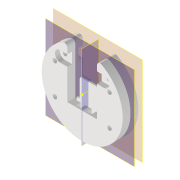
# Autodesk Inventor part: Matchboxscope_layer_ikealamp
Saved by Autodesk Inventor 2022 (Build 260153000, 153)
## iProperties
Created: 2022-04-02
Part Number: Matchboxscope_layer_ikealamp
Material: Generic
Document SubType Name: Modeling
Designer: Prakash Lab
Density: 1 g/cm^3
Appearance: Default
Author: Prakash Lab
Autodesk Inventor part; units mm, degrees
ref_plane "YZ Plane" through (0, 0, 0) normal (1, 0, 0) x (0, 1, 0)
ref_plane "XZ Plane" through (0, 0, 0) normal (0, 1, 0) x (-1, 0, 0)
ref_plane "XY Plane" through (0, 0, 0) normal (0, 0, 1) x (1, 0, 0)
ref_plane "Work Plane1" through (0, 0, 0) normal (0, 0, 1) x (1, 0, 0)
sketch "Sketch1" plane through (0, 0, 0) normal (0, 0, 1) x (1, 0, 0)
  circle A0 centre (0, 0) radius 25.9979 projected
  circle A1 centre (-9.4998, -11.0022) radius 2.6601 projected
  circle A2 centre (0.0001, -0.0022) radius 3.8801 projected
  circle A3 centre (0.0001, -0.0022) radius 6.7754 projected
  circle A4 centre (0.0001, -0.0022) radius 10
  point P0 (0, 0)
  dimension "d17" = 20
  constraints: 1 centre point, 1 coincident
  measures "d17" diameter of A4
extrude "Extrusion1" add sketch "Sketch1" along normal blind 10 contours A0 | A1 | A2 | A3 | A4
ref_plane "Arbeitsebene4" through (0, 0, 5) normal (0, 0, -1) x (-1, 0, 0)
sketch "Skizze22" plane through (0, 0, 10) normal (0, 0, 1) x (1, 0, 0)
  circle A0 centre (0, 0) radius 25.9979 projected
  line L0 (-9.5, 60.9958) -> (9.5, 60.9958)
  line L1 (9.5, 60.9958) -> (9.5, -9)
  line L2 (9.5, -9) -> (-9.5, -9)
  line L3 (-9.5, -9) -> (-9.5, 60.9958)
  line L4 (-9.5, 60.9958) -> (9.5, -9) construction
  line L5 (9.5, 60.9958) -> (-9.5, -9) construction
  point P0 (0, 0)
  point P1 (0, 25.9979)
  point P2 (2.05, -9)
  dimension "d82" = 19
  constraints: 12 end point, 2 midpoint, 2 parallel, 1 horizontal, 1 perpendicular, 1 point on line, 1 vertical alignment, 2 other
  measures "d82" distance of L1.end L2.end
extrude "Extrusion16" cut sketch "Skizze22" against normal blind 10 contours L1 L2 L3 A0 | A0 L3 L0 L1 picked at (-1.0778, 2.5987)
sketch "Skizze23" plane through (0, 0, 5) normal (0, 0, -1) x (-1, 0, 0)
  line L0 (-5.5222, 4.15) -> (-5.3125, 4.7) projected
  line L1 (-5.3125, 4.7) -> (5.3352, 4.7) projected
  line L2 (5.3352, 4.7) -> (5.5222, 4.15) projected
  line L3 (5.5222, 4.15) -> (5.7, 3.9722) projected
  line L4 (5.7, 3.9722) -> (5.7, -4) projected
  line L5 (4.85, -4) -> (5.7, -4) projected
  arc A0 (4.05, -3.2) -> (4.85, -4) centre (4.85, -3.2) ccw projected
  line L6 (4.05, -3.2) -> (4.05, 1.7) projected
  line L7 (4.05, 1.7) -> (2.85, 1.7) projected
  line L8 (2.85, -3.2) -> (2.85, 1.7) projected
  arc A1 (2.05, -4) -> (2.85, -3.2) centre (2.05, -3.2) ccw projected
  line L9 (-2.05, -4) -> (2.05, -4) projected
  arc A2 (-2.85, -3.2) -> (-2.05, -4) centre (-2.05, -3.2) ccw projected
  line L10 (-2.85, -3.2) -> (-2.85, 1.7) projected
  line L11 (-2.85, 1.7) -> (-4.05, 1.7) projected
  line L12 (-4.05, -3.2) -> (-4.05, 1.7) projected
  arc A3 (-4.85, -4) -> (-4.05, -3.2) centre (-4.85, -3.2) ccw projected
  line L13 (-5.7, -4) -> (-4.85, -4) projected
  line L14 (-5.7, -4) -> (-5.7, 3.9722) projected
  line L15 (-5.7, 3.9722) -> (-5.5222, 4.15) projected
  line L16 (5.7, -4) -> (5.7, -7) projected
  line L17 (5.7, -7) -> (7.5, -7) projected
  line L18 (7.5, -7) -> (7.5, -9) projected
  line L19 (7.5, -9) -> (4.85, -9) projected
  line L20 (4.85, -6) -> (4.85, -9) projected
  line L21 (4.85, -4) -> (4.85, -6) projected
  line L22 (4.85, -4) -> (5.7, -4) projected
  line L23 (-5.7, -7) -> (-5.7, -4) projected
  line L24 (-5.7, -4) -> (-4.85, -4) projected
  line L25 (-4.85, -4) -> (-4.85, -6) projected
  line L26 (-4.85, -6) -> (-4.85, -9) projected
  line L27 (-4.85, -9) -> (-7.5, -9) projected
  line L28 (-7.5, -9) -> (-7.5, -7) projected
  line L29 (-7.5, -7) -> (-5.7, -7) projected
  line L30 (-4.85, -9) -> (4.85, -9)
  constraints: 2 end point, 1 horizontal
extrude "Extrusion17" add sketch "Skizze23" along normal mid plane 1.9
sketch "Skizze24" plane through (0, 0, 5.95) normal (0, 0, -1) x (1, 0, 0)
  line L0 (2.85, 3.2) -> (2.85, -1.7) projected
  line L1 (2.85, -1.7) -> (4.05, -1.7) projected
  line L2 (4.05, 3.2) -> (4.05, -1.7) projected
  arc A0 (4.85, 4) -> (4.05, 3.2) centre (4.85, 3.2) ccw projected
  line L3 (4.85, 4) -> (4.85, 6) projected
  arc A1 (2.85, 3.2) -> (2.05, 4) centre (2.05, 3.2) ccw projected
  line L4 (2.05, 4) -> (2.05, 6) projected
  line L5 (4.85, 6) -> (4.85, 9) projected
  line L6 (2.05, 6) -> (2.05, 9) projected
  line L7 (9.5, 9) -> (-9.5, 9) projected
  line L8 (-2.05, 6) -> (-2.05, 9) projected
  line L9 (-4.85, 6) -> (-4.85, 9) projected
  line L10 (-2.15, 5.5641) -> (-2.15, 4)
  line L11 (-2.05, 4) -> (-2.05, 6) projected
  line L12 (-4.85, 4) -> (-4.85, 6) projected
  arc A2 (-4.05, 3.2) -> (-4.85, 4) centre (-4.85, 3.2) ccw projected
  arc A3 (-2.05, 4) -> (-2.85, 3.2) centre (-2.05, 3.2) ccw projected
  line L13 (-2.85, 3.2) -> (-2.85, -1.7) projected
  line L14 (-4.05, 3.2) -> (-4.05, -1.7) projected
  line L15 (-4.05, -1.7) -> (-2.85, -1.7) projected
  constraints: 2 end point, 1 vertical, 2 other
extrude "Extrusion18" cut sketch "Skizze24" along normal blind 1
sketch "Skizze25" plane through (-9.5, -9, 10) normal (0, 1, 0) x (1, 0, 0)
  line L0 (14.4863, 5) -> (11.4863, 5)
  line L1 (11.4863, 5) -> (11.4863, 2)
  line L2 (11.4863, 2) -> (14.4863, 2)
  line L3 (14.4863, 2) -> (14.4863, 5)
  line L4 (7.4938, 5) -> (4.4938, 5)
  line L5 (4.4938, 5) -> (4.4938, 2)
  line L6 (4.4938, 2) -> (7.4938, 2)
  line L7 (7.4938, 2) -> (7.4938, 5)
  line L8 (19, 0) -> (0, 0) projected
  line L9 (19, 0) -> (19, 10) projected
  line L10 (0, 10) -> (19, 10) projected
  line L11 (0, 0) -> (0, 10) projected
  point P0 (9.5, 10)
  dimension "d90" = 3
  dimension "d91" = 3
  dimension "d92" = 3
  dimension "d93" = 3
  constraints: 16 end point, 4 parallel, 2 horizontal, 2 perpendicular, 1 point on line
  measures "d90" distance of L2.end L1.end
  measures "d91" distance of L1.end L0.end
  measures "d92" distance of L6.end L5.end
  measures "d93" distance of L5.end L4.end
extrude "Extrusion19" cut sketch "Skizze25" against normal through all contours L3 L2 L1 L0 | L7 L6 L5 L4
sketch "Skizze26" plane through (0, 0, 10) normal (0, 0, 1) x (1, 0, 0)
  line L0 (9.5, 24.2) -> (9.5, -9) projected
  line L1 (9.5, -9) -> (-9.5, -9) projected
  line L2 (-9.5, -9) -> (-9.5, 24.2) projected
  arc A0 (-9.5, 24.2) -> (9.5, 24.2) centre (0, 0) ccw projected
  line L3 (-14, 14.1304) -> (14, 14.1304) construction
  line L4 (-14, 10.6304) -> (14, 10.6304)
  line L5 (14, 17.6304) -> (-14, 17.6304)
  arc A1 (-14, 17.6304) -> (-14, 10.6304) centre (-14, 14.1304) ccw
  arc A2 (14, 10.6304) -> (14, 17.6304) centre (14, 14.1304) ccw
  point P0 (0, 0)
  point P1 (0, 14.1304)
  dimension "d96" = 14
  dimension "d97" = 7
  constraints: 8 end point, 4 point on circle, 4 tangent, 2 centre point, 1 horizontal, 1 midpoint, 1 parallel
  measures "d96" distance of point (0, 14.13) L3.end
  measures "d97" diameter of A2
extrude "Extrusion20" cut sketch "Skizze26" against normal blind 3 contours L5 A2 L4 L0 | L0 L4 L2 L5 | L2 L4 A1 L5
sketch "Skizze27" plane through (0, 0, 0) normal (0, 0, -1) x (-1, 0, 0)
  line L0 (-9.5, 10.6304) -> (-9.5, 17.6304) projected
  line L1 (-14, 10.6304) -> (-9.5, 10.6304) projected
  arc A0 (-14, 17.6304) -> (-14, 10.6304) centre (-14, 14.1304) ccw projected
  line L2 (-9.5, 17.6304) -> (-14, 17.6304) projected
  line L3 (9.5, 17.6304) -> (9.5, 10.6304) projected
  line L4 (14, 17.6304) -> (9.5, 17.6304) projected
  arc A1 (14, 10.6304) -> (14, 17.6304) centre (14, 14.1304) ccw projected
  line L5 (9.5, 10.6304) -> (14, 10.6304) projected
  point P0 (0, 0)
extrude "Extrusion21" cut sketch "Skizze27" against normal blind 3
sketch "Skizze28" plane through (0, 0, 0) normal (0, 0, -1) x (-1, 0, 0)
  arc A0 (-14, 17.6304) -> (-14, 10.6304) centre (-14, 14.1304) ccw projected
  arc A1 (14, 10.6304) -> (14, 17.6304) centre (14, 14.1304) ccw projected
  circle A2 centre (-14, 14.1304) radius 1.4
  circle A3 centre (14, 14.1304) radius 1.4
  point P0 (0, 0)
  dimension "d102" = 2.8
  dimension "d103" = 2.8
  constraints: 2 centre point, 2 coincident
  measures "d102" diameter of A2
  measures "d103" diameter of A3
extrude "Extrusion22" cut sketch "Skizze28" against normal through all
fillet "Rundung3" radius 2 2 edges at (9.5, 24.2, 5) (-9.5, 24.2, 5)
ref_plane "Arbeitsebene5" through (0, 0, 5) normal (0, 0, 1) x (1, 0, 0)
sketch "Skizze29" plane through (0, 0, 10) normal (0, 0, 1) x (1, 0, 0)
  point P0 (0, 0)
sketch "Skizze30" plane through (0, 0, 10) normal (0, 0, 1) x (1, 0, 0)
  circle A0 centre (-17.4978, -9.9998) radius 1.3999 projected
  circle A1 centre (-17.4979, 10.0001) radius 1.4 projected
  circle A2 centre (17.5021, 10.0001) radius 1.4 projected
  circle A3 centre (17.5021, -9.9999) radius 1.4001 projected
  circle A4 centre (0.0022, 0.0001) radius 3.95 projected
  circle A5 centre (11.0022, -9.4998) radius 2.6601 projected
  line L0 (19.0307, -17.7122) -> (18.4312, -14.7304) projected
  line L1 (18.4312, -14.7304) -> (15.4222, -13.716) projected
  line L2 (15.4222, -13.716) -> (13.0391, -15.8146) projected
  line L3 (13.0391, -15.8146) -> (13.6651, -18.9277) projected
  line L4 (13.6651, -18.9277) -> (16.6741, -19.9422) projected
  line L5 (16.6741, -19.9422) -> (17.7641, -18.9823) projected
  arc A6 (7.7254, -24.8235) -> (17.7641, -18.9823) centre (0, 0) ccw projected
  arc A7 (6.496, -23.8502) -> (7.7254, -24.8235) centre (7.496, -23.8502) ccw projected
  line L6 (6.496, -23.8502) -> (6.496, -17.7002) projected
  arc A8 (6.496, -17.7002) -> (4.496, -15.7002) centre (4.496, -17.7002) ccw projected
  line L7 (4.496, -15.7002) -> (-3.4917, -15.7002) projected
  arc A9 (-3.4917, -15.7002) -> (-5.4917, -17.7002) centre (-3.4917, -17.7002) ccw projected
  line L8 (-5.4917, -17.7002) -> (-5.4917, -24.1417) projected
  arc A10 (-6.6998, -25.1198) -> (-5.4917, -24.1417) centre (-6.4917, -24.1417) ccw projected
  arc A11 (-25.545, 4.8315) -> (-6.6998, -25.1198) centre (0, 0) ccw projected
  line L9 (-25.545, 4.8315) -> (-24.0265, 3.1166) projected
  line L10 (-24.0265, 3.1166) -> (-20.9151, 3.751) projected
  line L11 (-20.9151, 3.751) -> (-19.9088, 6.7628) projected
  line L12 (-19.9088, 6.7628) -> (-22.0139, 9.1401) projected
  line L13 (-22.0139, 9.1401) -> (-24.5243, 8.6283) projected
  arc A12 (-9.6986, 24.1211) -> (-24.5243, 8.6283) centre (0, 0) ccw projected
  line L14 (-9.6986, 24.1211) -> (-10.2078, 21.7325) projected
  line L15 (-10.2078, 21.7325) -> (-7.8493, 19.6063) projected
  line L16 (-7.8493, 19.6063) -> (-4.8287, 20.5857) projected
  line L17 (-4.8287, 20.5857) -> (-4.1666, 23.6914) projected
  line L18 (-4.1666, 23.6914) -> (-5.9577, 25.306) projected
  arc A13 (19.0307, -17.7122) -> (-5.9577, 25.306) centre (0, 0) ccw projected
  point P0 (0, 0)
hole "Bohrung2" at (-17.4978, -9.9998, 10) at (-17.4979, 10.0001, 10) at (17.5021, -9.9999, 10) at (17.5021, 10.0001, 10) direction (0, 0, -1) diameter 2.9 depth 7 tip angle 118
ref_plane "Arbeitsebene6" through (0, -9, 0) normal (-1, 0, 0) x (0, 0, 1)
body "Solid1"
